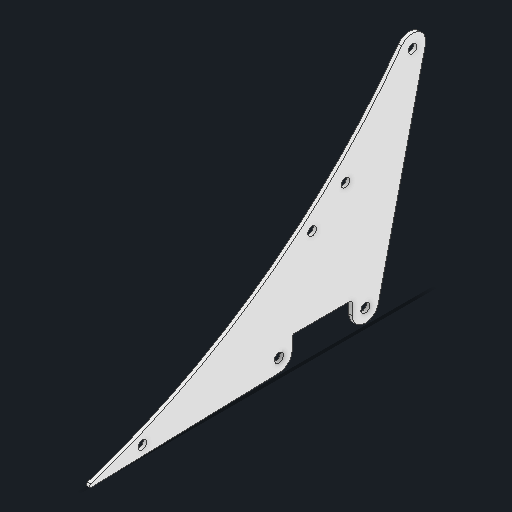
# Autodesk Inventor part: Ramp V2
Saved by Autodesk Inventor 2025.1 (Build 291241000, 241)
## iProperties
Created: 2024-10-13
Part Number: Ramp V2
Material: Acetal Resin, White
Document SubType Name: Sheet Metal
Designer: Averey Ku
Density: 1.425 g/cm^3
Appearance: Smooth - White
Mass: 12.8393 g
Surface Area: 122.133 cm^2
Volume: 9.01001 cm^3
Flat Pattern Width: 13.2736 cm
Flat Pattern Length: 14.3407 cm
Flat Pattern Area: 190.353 cm^2
Sheet Metal Rule: Default_mm
Sheet Metal Width: 5.226 in
Sheet Metal Length: 5.646 in
Sheet Metal Area: 29.505 in^2
Author: Averey Ku
Autodesk Inventor part; units mm, degrees
ref_plane "YZ Plane" through (0, 0, 0) normal (1, 0, 0) x (0, 1, 0)
ref_plane "XZ Plane" through (0, 0, 0) normal (0, 1, 0) x (-1, 0, 0)
ref_plane "XY Plane" through (0, 0, 0) normal (0, 0, 1) x (1, 0, 0)
sketch "main" plane through (0, 0, 0) normal (0, 0, 1) x (1, 0, 0)
  circle A0 centre (-191.7635, 49.9495) radius 2.1844
  circle A1 centre (-95.8324, -13.8772) radius 2.1
  arc A2 (-99.5462, -18.9735) -> (-92.0695, -8.7075) centre (-95.8064, -13.8415) ccw
  arc A3 (-198.1111, 49.7757) -> (-191.7635, 43.5995) centre (-191.7635, 49.9495) ccw
  line L0 (-200.5697, 139.5363) -> (-198.1111, 49.7757)
  arc A4 (-199.0195, 139.7975) -> (-92.0695, -8.7075) centre (80.274, 228.1743) ccw
  circle A5 centre (-195.1368, 115.1254) radius 2.0828
  line L1 (-191.7635, 43.5995) -> (-186.2072, 43.5995)
  arc A6 (-199.0195, 139.7975) -> (-200.5697, 139.5363) centre (-199.7762, 139.5581) ccw
  circle A7 centre (-135.2274, 18.1995) radius 2.0828
  circle A8 centre (-191.7635, 8.6745) radius 2.1844
  arc A9 (-191.7635, 15.0245) -> (-193.2141, 2.4924) centre (-191.7635, 8.6745) ccw
  line L2 (-185.4135, 15.8183) -> (-185.4135, 42.8058)
  line L3 (-191.7635, 15.0245) -> (-186.2072, 15.0245)
  arc A10 (-185.4135, 42.8058) -> (-186.2072, 43.5995) centre (-186.2072, 42.8058) ccw
  arc A11 (-186.2072, 15.0245) -> (-185.4135, 15.8183) centre (-186.2072, 15.8183) ccw
  line L4 (-193.2141, 2.4924) -> (-97.2571, -20.0236)
  point P0 (1.1251, 9.7944)
  point P1 (-200.7302, 145.398)
  dimension "d7" = 12.7
  dimension "d8" = 4.1656
  dimension "d9" = 6.35
  dimension "d11" = 0.7937
  dimension "d13" = 4.1656
  dimension "d15" = 12.7
  dimension "d16" = 0.7937
  measures "d7" diameter of A3
  measures "d8" diameter of A5
  measures "d9" radius of A2
  measures "d11" radius of A6
  measures "d13" diameter of A7
  measures "d15" diameter of A9
  measures "d16" radius of A10
sketch "Sketch1" plane through (0, 0, 0) normal (1, 0, 0) x (0, 1, 0)
  circle A0 centre (44.45, -15.875) radius 2.0955
  circle A1 centre (0, 0) radius 2.1844
  circle A2 centre (95.9311, -63.8268) radius 2.1
  arc A3 (92.2173, -68.923) -> (99.694, -58.6571) centre (95.9571, -63.7911) ccw
  arc A4 (-6.3476, -0.1739) -> (0, -6.35) centre (0, 0) ccw
  line L0 (-8.8062, 89.5868) -> (-6.3476, -0.1739)
  arc A5 (-7.256, 89.848) -> (99.694, -58.6571) centre (272.0375, 178.2247) ccw
  circle A6 centre (-3.3733, 65.1759) radius 2.0828
  line L1 (0, -6.35) -> (5.5563, -6.35)
  arc A7 (-7.256, 89.848) -> (-8.8062, 89.5868) centre (-8.0127, 89.6085) ccw
  circle A8 centre (56.5361, -31.75) radius 2.0828
  circle A9 centre (0, -41.275) radius 2.1844
  arc A10 (0, -34.925) -> (-1.4506, -47.4571) centre (0, -41.275) ccw
  line L2 (6.35, -34.1313) -> (6.35, -7.1438)
  line L3 (0, -34.925) -> (5.5563, -34.925)
  arc A11 (6.35, -7.1438) -> (5.5563, -6.35) centre (5.5563, -7.1437) ccw
  arc A12 (5.5563, -34.925) -> (6.35, -34.1313) centre (5.5563, -34.1313) ccw
  line L4 (-1.4506, -47.4571) -> (94.5064, -69.9732)
  dimension "d18" = 4.191
  constraints: 1 centre point, 1 other
  measures "d18" diameter of A0
extrude "Extrusion1" add sketch "Sketch1" along normal blind 1.5875
equation "\"BendRadius\" = Thickness"
equation "\"BendReliefWidth\" = Thickness"
equation "\"BendReliefDepth\" = 0.5 * Thickness"
equation "\"CornerReliefSize\" = 4 * Thickness"
equation "\"MinimumRemnant\" = 2 * Thickness"
equation "\"TransitionRadius\" = BendRadius"
equation "\"JacobiRadiusSize\" = BendRadius"
equation "\"GapSize\" = Thickness"
equation "\"Thickness\" = 1.5875"
body "Solid1"
